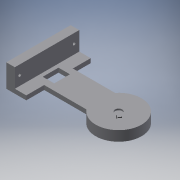
# Autodesk Inventor part: arm
Saved by Autodesk Inventor 2017 (Build 210142000, 142)
## iProperties
Created: 2020-01-31
Part Number: arm
Material: Generic
Document SubType Name: Modeling
Designer: blep
Density: 1 g/cm^3
Appearance: Default
Author: blep
Autodesk Inventor part; units mm, degrees
ref_plane "YZ Plane" through (0, 0, 0) normal (1, 0, 0) x (0, 1, 0)
ref_plane "XZ Plane" through (0, 0, 0) normal (0, 1, 0) x (-1, 0, 0)
ref_plane "XY Plane" through (0, 0, 0) normal (0, 0, 1) x (1, 0, 0)
sketch "Sketch1" plane through (0, 0, 0) normal (0, 0, 1) x (1, 0, 0)
  line L0 (-15.25, 6.5) -> (-15.25, -6.5) construction
  line L1 (18.75, 6.5) -> (-15.25, 6.5) construction
  line L2 (18.75, -6.5) -> (18.75, 6.5) construction
  line L3 (-15.25, -6.5) -> (18.75, -6.5) construction
  line L4 (9.8054, 8.5) -> (19.75, 8.5) construction
  arc A0 (9.8054, 8.5) -> (9.8054, -8.5) centre (-3.75, 0) ccw construction
  line L5 (19.75, -8.5) -> (9.8054, -8.5) construction
  line L6 (19.75, 8.5) -> (19.75, -8.5) construction
  circle A1 centre (-3.75, 0) radius 16
  point P0 (0, 0)
  constraints: 1 centre point, 1 coincident, 1 concentric
extrude "Extrusion1" add sketch "Sketch1" along normal blind 7
sketch "Sketch4" plane through (-3.75, 0, 7) normal (0, 0, 1) x (1, 0, 0)
  line L0 (0, 0) -> (-50, 0) construction
  line L1 (0, 10) -> (-50, 10)
  line L2 (-50, -10) -> (0, -10)
  arc A0 (0, -10) -> (0, 10) centre (0, 0) ccw
  arc A1 (-50, 10) -> (-50, -10) centre (-50, 0) ccw
  point P0 (3.75, 0)
  point P1 (-25, 0)
  dimension "d6" = 50
  dimension "d7" = 10
  constraints: 8 end point, 4 point on circle, 4 tangent, 2 centre point, 1 horizontal, 1 midpoint, 1 parallel
  measures "d6" distance of L0.start L0.end
  measures "d7" radius of A1
extrude "Extrusion3" add sketch "Sketch4" against normal blind 3
sketch "Sketch5" plane through (0, 0, 7) normal (0, 0, 1) x (1, 0, 0)
  arc A0 (-53.75, 10) -> (-53.75, -10) centre (-53.75, 0) ccw construction
  line L0 (-53.75, -10) -> (-16.24, -10) construction
  line L1 (-16.24, 10) -> (-53.75, 10) construction
  line L2 (-45.75, -22.5) -> (-61.75, -22.5)
  line L3 (-61.75, -22.5) -> (-61.75, 22.5)
  line L4 (-61.75, 22.5) -> (-45.75, 22.5)
  line L5 (-45.75, 22.5) -> (-45.75, -22.5)
  line L6 (-61.75, -22.5) -> (-45.75, 22.5) construction
  line L7 (-45.75, -22.5) -> (-61.75, 22.5) construction
  line L8 (-77.75, -22.5) -> (-61.75, -22.5)
  line L9 (-61.75, -22.5) -> (-61.75, 22.5)
  line L10 (-61.75, 22.5) -> (-77.75, 22.5)
  line L11 (-77.75, 22.5) -> (-77.75, -22.5)
  point P0 (0, 0)
  dimension "d10" = 45
  dimension "d11" = 16
  dimension "d12" = 16
  constraints: 20 end point, 4 parallel, 3 collinear, 2 horizontal, 2 perpendicular, 1 coincident, 1 midpoint
  measures "d10" distance of L2.end L3.end
  measures "d11" distance of L2.start L2.end
  measures "d12" distance of L8.start L8.end
extrude "Extrusion4" cut sketch "Sketch5" against normal blind 3 contours L8 L11 L10 L3
extrude "Extrusion5" add sketch "Sketch5" against normal blind 3 contours L2 L3 L4 L5
sketch "Sketch6" plane through (0, 0, 7) normal (0, 0, 1) x (1, 0, 0)
  line L0 (-53.75, -22.5) -> (-61.75, -22.5)
  line L1 (-61.75, -22.5) -> (-61.75, 22.5)
  line L2 (-61.75, 22.5) -> (-53.75, 22.5)
  line L3 (-53.75, 22.5) -> (-53.75, -22.5)
  line L4 (-61.75, -22.5) -> (-61.75, 22.5) construction
  line L5 (-45.75, -22.5) -> (-61.75, -22.5) projected
  line L6 (-61.75, 22.5) -> (-45.75, 22.5) projected
  point P0 (0, 0)
  dimension "d17" = 8
  constraints: 8 end point, 3 collinear, 2 parallel, 1 horizontal, 1 perpendicular
  measures "d17" distance between parallel lines of L1 L3
extrude "Extrusion6" add sketch "Sketch6" along normal blind 13
sketch "Sketch7" plane through (0, 0, 7) normal (0, 0, 1) x (1, 0, 0)
  line L0 (-43.25, -5.5) -> (-51.25, -5.5)
  line L1 (-51.25, -5.5) -> (-51.25, 5.5)
  line L2 (-51.25, 5.5) -> (-43.25, 5.5)
  line L3 (-43.25, 5.5) -> (-43.25, -5.5)
  line L4 (-53.75, -22.5) -> (-53.75, 22.5) projected
  line L5 (-53.75, -22.5) -> (-51.25, -5.5) construction
  line L6 (-51.25, 5.5) -> (-53.75, 22.5) construction
  point P0 (0, 0)
  dimension "d20" = 2.5
  dimension "d21" = 8
  dimension "d22" = 11
  constraints: 12 end point, 2 parallel, 1 equal length, 1 horizontal, 1 perpendicular
  measures "d20" distance between parallel lines of L4 L1
  measures "d21" distance of L0.start L0.end
  measures "d22" distance of L0.end L1.end
extrude "Extrusion7" cut sketch "Sketch7" against normal through all
sketch "Sketch8" plane through (0, 0, 20) normal (0, 0, 1) x (1, 0, 0)
  line L0 (-59.75, -22.5) -> (-61.75, -22.5)
  line L1 (-61.75, -22.5) -> (-61.75, 22.5)
  line L2 (-61.75, 22.5) -> (-59.75, 22.5)
  line L3 (-59.75, 22.5) -> (-59.75, -22.5)
  line L4 (-61.75, 22.5) -> (-61.75, -22.5) projected
  line L5 (-61.75, -22.5) -> (-53.75, -22.5) projected
  line L6 (-53.75, 22.5) -> (-61.75, 22.5) projected
  point P0 (0, 0)
  dimension "d25" = 2
  constraints: 8 end point, 3 collinear, 2 parallel, 1 horizontal, 1 perpendicular
  measures "d25" distance of L0.start L0.end
extrude "Extrusion8" cut sketch "Sketch8" against normal through all
ref_plane "Work Plane1" through (-3.75, 0, 3.5) normal (0, 0, -1) x (-1, 0, 0)
sketch "Sketch12" plane through (0, 0, 7) normal (0, 0, 1) x (1, 0, 0)
  arc A0 (-16.24, -10) -> (-16.24, 10) centre (-3.75, 0) ccw projected
  circle A1 centre (-3.75, 0) radius 3
  point P0 (0, 0)
  dimension "d46" = 6
  constraints: 1 centre point, 1 coincident
  measures "d46" diameter of A1
extrude "Extrusion11" cut sketch "Sketch12" against normal through all
sketch "Sketch13" plane through (-53.75, -22.5, 7) normal (1, 0, 0) x (0, 0, -1)
  line L0 (0, 45) -> (-13, 45) projected
  line L1 (0, 0) -> (-13, 0) projected
  line L2 (-13, 0) -> (-13, 45) construction
  line L3 (0, 12.5) -> (0, 0) construction
  line L4 (0, 45) -> (0, 32.5) construction
  line L5 (-6.5, 3.5) -> (-13, 3.5) construction
  line L6 (-6.5, 3.5) -> (0, 3.5) construction
  line L7 (-6.5, 41.5) -> (-13, 41.5) construction
  line L8 (-6.5, 41.5) -> (0, 41.5) construction
  point P0 (7, 22.5)
  dimension "d37" = 3.5
  dimension "d38" = 3.5
  constraints: 8 end point, 5 point on line, 2 collinear, 2 perpendicular, 1 horizontal
  measures "d37" distance from line of L0 L7.start
  measures "d38" distance from line of L1 L5.start
hole "Hole1" at (-53.75, -19, 13.5) at (-53.75, 19, 13.5) direction (-1, 0, 0) diameter 2 depth 5 tip angle 118
sketch "Sketch14" plane through (-3.75, 0, 0) normal (0, 0, -1) x (-1, 0, 0)
  circle A0 centre (0, 0) radius 7
  point P0 (-3.75, 0)
  dimension "d47" = 14
  constraints: 1 centre point
  measures "d47" diameter of A0
extrude "Extrusion12" cut sketch "Sketch14" against normal blind 5
equation "\"d38\" = d37"
body "Solid1"
